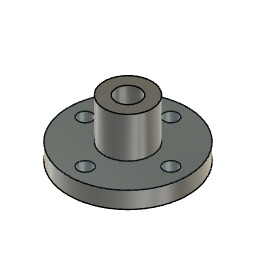
shaftholder (Autodesk Fusion 360 design; units mm, degrees)
Autodesk Fusion 360 part; units mm, degrees
note: some values were not read from the file. Set by a fixed rule: which sketch regions a step uses.
sketch "スケッチ1" plane through (0, 0, 0) normal (0, 0, 1) x (1, 0, 0)
  circle A0 centre (0, 0) radius 12.5
  dimension "d1" = 25
  constraint coincident A0.centre origin
  measures "d1" diameter of A0
extrude "押し出し1" add sketch "スケッチ1" along normal blind 3.5
sketch "スケッチ2" plane through (0, 0, 3.5) normal (0, 0, 1) x (-1, 0, 0)
  circle A0 centre (0, 0) radius 12.5
  circle A1 centre (0, 0) radius 5
  dimension "d4" = 10
  constraint coincident A0.centre A1.centre
  measures "d4" diameter of A1
extrude "押し出し2" add sketch "スケッチ2" along normal blind 8.5 contours A1
sketch "スケッチ3" plane through (0, 0, 12) normal (0, 0, 1) x (-1, 0, 0)
  circle A0 centre (0, 0) radius 5
  circle A1 centre (0, 0) radius 2.5
  dimension "d7" = 5
  constraint coincident A0.centre A1.centre
  measures "d7" diameter of A1
extrude "押し出し3" cut sketch "スケッチ3" against normal blind 12 contours A1
sketch "スケッチ4" plane through (0, 0, 3.5) normal (0, 0, 1) x (-1, 0, 0)
  circle A0 centre (0, 0) radius 5
  circle A1 centre (0, 0) radius 12.5
  line L0 (12.5, 0) -> (-12.5, 0)
  line L1 (0, 0) -> (-9, 0)
  line L2 (0, 0) -> (9, 0)
  circle A2 centre (-9, 0) radius 1.5
  circle A3 centre (0, -9) radius 1.5
  circle A4 centre (9, 0) radius 1.5
  circle A5 centre (0, 9) radius 1.5
  dimension "d10" = 25
  dimension "d11" = 9
  dimension "d12" = 9
  dimension "d13" = 3
  dimension "d15" = 360
  constraint coincident A1 L0.start
  constraint horizontal L0
  constraint coincident A0.centre A1.centre
  constraint coincident L0 L1.end
  constraint parallel L0 L1
  constraint parallel L0 L2
  constraint coincident L1.end A2.centre
  measures "d10" distance of L0.start L0.end
  measures "d11" distance of A0.centre L1.end
  measures "d12" distance of A0.centre L2.end
  measures "d13" diameter of A2
extrude "押し出し4" cut sketch "スケッチ4" against normal blind 3.5 contours L0 L2 A4 | L0 L2 A4 | L0 L1 A2 | L0 L1 A2 | A3 | A5
sketch "スケッチ5" plane through (0, 0, 3.5) normal (0, 0, 1) x (-1, 0, 0)
  circle A0 centre (0, 9) radius 1.5
  circle A1 centre (9, 0) radius 1.5
  circle A2 centre (-9, 0) radius 1.5
  circle A3 centre (0, -9) radius 1.5
  circle A4 centre (0, 0) radius 5
  circle A5 centre (0, 0) radius 12.5
